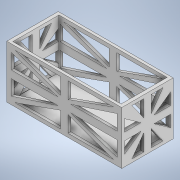
# Autodesk Inventor part: BatteryHolder
Saved by Autodesk Inventor 2022 (Build 260153000, 153)
## iProperties
Created: 2022-02-22
Part Number: BatteryHolder
Material: Generic
Document SubType Name: Modeling
Designer: merky
Density: 1 g/cm^3
Appearance: Default
Author: merky
Autodesk Inventor part; units mm, degrees
ref_plane "YZ Plane" through (0, 0, 0) normal (1, 0, 0) x (0, 1, 0)
ref_plane "XZ Plane" through (0, 0, 0) normal (0, 1, 0) x (-1, 0, 0)
ref_plane "XY Plane" through (0, 0, 0) normal (0, 0, 1) x (1, 0, 0)
sketch "Sketch1" plane through (0, 0, 0) normal (0, 1, 0) x (-1, 0, 0)
  line L0 (-90.805, 38.735) -> (90.805, 38.735)
  line L1 (90.805, 38.735) -> (90.805, -38.735)
  line L2 (90.805, -38.735) -> (-90.805, -38.735)
  line L3 (-90.805, -38.735) -> (-90.805, 38.735)
  line L4 (-90.805, 38.735) -> (90.805, -38.735) construction
  line L5 (90.805, 38.735) -> (-90.805, -38.735) construction
  line L6 (96.52, 43.18) -> (-96.52, 43.18)
  line L7 (-96.52, 43.18) -> (-96.52, -43.18)
  line L8 (-96.52, -43.18) -> (96.52, -43.18)
  line L9 (96.52, -43.18) -> (96.52, 43.18)
  line L10 (96.52, 43.18) -> (-96.52, -43.18) construction
  line L11 (-96.52, 43.18) -> (96.52, -43.18) construction
  point P0 (0, 0)
  dimension "d0" = 181.61
  dimension "d1" = 77.47
  dimension "d2" = 193.04
  dimension "d3" = 86.36
  constraints: 24 end point, 4 midpoint, 4 parallel, 2 horizontal, 2 perpendicular
  measures "d0" distance of L1.end L2.end
  measures "d1" distance of L0.end L1.end
  measures "d2" distance of L8.end L7.end
  measures "d3" distance of L7.end L6.end
extrude "Extrusion1" add sketch "Sketch1" against normal blind 5.08 contours L0 L1 L2 L3 | L9 L8 L7 L6
extrude "Extrusion2" add sketch "Sketch1" along normal blind 83.566
sketch "Sketch2" plane through (-96.52, -5.08, 43.18) normal (0, 0, 1) x (1, 0, 0)
  line L0 (187.325, 88.646) -> (5.715, 88.646) projected
  line L1 (193.04, 88.646) -> (193.04, 0) projected
  line L2 (7.62, 82.423) -> (185.42, 82.423)
  line L3 (185.42, 82.423) -> (185.42, 6.223)
  line L4 (185.42, 6.223) -> (7.62, 6.223)
  line L5 (7.62, 6.223) -> (7.62, 82.423)
  line L6 (185.42, 50.673) -> (185.42, 37.973)
  line L7 (7.62, 37.973) -> (7.62, 50.673)
  line L8 (90.17, 82.423) -> (102.87, 82.423)
  line L9 (102.87, 6.223) -> (90.17, 6.223)
  line L10 (7.62, 50.673) -> (85.5215, 50.673)
  line L11 (107.5185, 50.673) -> (185.42, 50.673)
  line L12 (90.17, 6.223) -> (90.17, 33.3245)
  line L13 (90.17, 55.3215) -> (90.17, 82.423)
  line L14 (185.42, 37.973) -> (107.5185, 37.973)
  line L15 (85.5215, 37.973) -> (7.62, 37.973)
  line L16 (102.87, 82.423) -> (102.87, 55.3215)
  line L17 (102.87, 33.3245) -> (102.87, 6.223)
  arc A0 (90.17, 55.3215) -> (85.5215, 50.673) centre (96.52, 44.323) ccw
  arc A1 (107.5185, 50.673) -> (102.87, 55.3215) centre (96.52, 44.323) ccw
  arc A2 (85.5215, 37.973) -> (90.17, 33.3245) centre (96.52, 44.323) ccw
  arc A3 (102.87, 33.3245) -> (107.5185, 37.973) centre (96.52, 44.323) ccw
  line L18 (7.62, 82.423) -> (13.97, 82.423)
  line L19 (13.97, 82.423) -> (13.97, 76.073)
  line L20 (13.97, 76.073) -> (7.62, 76.073)
  line L21 (7.62, 76.073) -> (7.62, 82.423)
  line L22 (185.42, 82.423) -> (179.07, 82.423)
  line L23 (179.07, 82.423) -> (179.07, 76.073)
  line L24 (179.07, 76.073) -> (185.42, 76.073)
  line L25 (185.42, 76.073) -> (185.42, 82.423)
  line L26 (185.42, 6.223) -> (179.07, 6.223)
  line L27 (179.07, 6.223) -> (179.07, 12.573)
  line L28 (179.07, 12.573) -> (185.42, 12.573)
  line L29 (185.42, 12.573) -> (185.42, 6.223)
  line L30 (7.62, 6.223) -> (13.97, 6.223)
  line L31 (13.97, 6.223) -> (13.97, 12.573)
  line L32 (13.97, 12.573) -> (7.62, 12.573)
  line L33 (7.62, 12.573) -> (7.62, 6.223)
  line L34 (13.97, 6.223) -> (90.17, 33.3245)
  line L35 (85.5215, 37.973) -> (7.62, 12.573)
  line L36 (85.5215, 50.673) -> (7.62, 76.073)
  line L37 (13.97, 82.423) -> (90.17, 55.3215)
  line L38 (102.87, 55.3215) -> (179.07, 82.423)
  line L39 (185.42, 76.073) -> (107.5185, 50.673)
  line L40 (107.5185, 37.973) -> (185.42, 12.573)
  line L41 (179.07, 6.223) -> (102.87, 33.3245)
  point P0 (96.52, 5.08)
  point P1 (96.52, 88.646)
  point P2 (193.04, 44.323)
  point P3 (13.97, 82.423)
  point P4 (13.97, 6.223)
  dimension "d8" = 177.8
  dimension "d9" = 76.2
  dimension "d11" = 12.7
  dimension "d12" = 12.7
  dimension "d13" = 6.35
  dimension "d14" = 6.35
  dimension "d15" = 6.35
  dimension "d16" = 6.35
  dimension "d17" = 6.35
  dimension "d18" = 6.35
  dimension "d19" = 6.35
  dimension "d20" = 6.35
  constraints: 80 end point, 24 parallel, 9 perpendicular, 8 horizontal, 8 point on circle, 4 centre point, 2 midpoint, 2 point on line, 1 coincident
  measures "d8" distance of L3.end L4.end
  measures "d9" distance of L2.end L3.end
  measures "d11" distance of L6.start L6.end
  measures "d12" distance of L9.start L9.end
  measures "d13" distance of L19.end L20.end
  measures "d14" distance of L18.end L19.end
  measures "d15" distance of L24.end L23.end
  measures "d16" distance of L23.end L22.end
  measures "d17" distance of L27.end L28.end
  measures "d18" distance of L26.end L27.end
  measures "d19" distance of L32.end L31.end
  measures "d20" distance of L31.end L30.end
extrude "Extrusion3" cut sketch "Sketch2" against normal through all contours L2 L13 L37 | L36 L10 L5 | L2 L38 L16 | L15 L35 L5 | L39 L3 L11 | L12 L4 L34 | L3 L40 L14 | L17 L41 L4
sketch "Sketch3" plane through (96.52, -5.08, 43.18) normal (1, 0, 0) x (0, 0, -1)
  line L0 (81.915, 88.646) -> (4.445, 88.646) projected
  line L1 (86.36, 0) -> (86.36, 88.646) projected
  line L2 (81.915, 5.08) -> (81.915, 88.646) projected
  line L3 (4.445, 83.058) -> (81.915, 83.058)
  line L4 (81.915, 83.058) -> (81.915, 5.588)
  line L5 (81.915, 5.588) -> (4.445, 5.588)
  line L6 (4.445, 5.588) -> (4.445, 83.058)
  circle A0 centre (43.18, 44.323) radius 12.7
  line L7 (81.915, 50.673) -> (81.915, 37.973)
  line L8 (4.445, 37.973) -> (4.445, 50.673)
  line L9 (36.83, 83.058) -> (49.53, 83.058)
  line L10 (49.53, 5.588) -> (36.83, 5.588)
  line L11 (4.445, 50.673) -> (32.1815, 50.673)
  line L12 (54.1785, 50.673) -> (81.915, 50.673)
  line L13 (36.83, 5.588) -> (36.83, 33.3245)
  line L14 (36.83, 55.3215) -> (36.83, 83.058)
  line L15 (81.915, 37.973) -> (54.1785, 37.973)
  line L16 (32.1815, 37.973) -> (4.445, 37.973)
  line L17 (49.53, 83.058) -> (49.53, 55.3215)
  line L18 (49.53, 33.3245) -> (49.53, 5.588)
  line L19 (4.445, 83.058) -> (17.145, 83.058)
  line L20 (17.145, 83.058) -> (17.145, 70.358)
  line L21 (17.145, 70.358) -> (4.445, 70.358)
  line L22 (4.445, 70.358) -> (4.445, 83.058)
  line L23 (81.915, 83.058) -> (69.215, 83.058)
  line L24 (69.215, 83.058) -> (69.215, 70.358)
  line L25 (69.215, 70.358) -> (81.915, 70.358)
  line L26 (81.915, 70.358) -> (81.915, 83.058)
  line L27 (4.445, 5.588) -> (17.145, 5.588)
  line L28 (17.145, 5.588) -> (17.145, 18.288)
  line L29 (17.145, 18.288) -> (4.445, 18.288)
  line L30 (4.445, 18.288) -> (4.445, 5.588)
  line L31 (81.915, 5.588) -> (69.215, 5.588)
  line L32 (69.215, 5.588) -> (69.215, 18.288)
  line L33 (69.215, 18.288) -> (81.915, 18.288)
  line L34 (81.915, 18.288) -> (81.915, 5.588)
  line L35 (17.145, 5.588) -> (36.83, 33.3245)
  line L36 (32.1815, 37.973) -> (4.445, 18.288)
  line L37 (69.215, 5.588) -> (49.53, 33.3245)
  line L38 (54.1785, 37.973) -> (81.915, 18.288)
  line L39 (49.53, 55.3215) -> (69.215, 83.058)
  line L40 (54.1785, 50.673) -> (81.915, 70.358)
  line L41 (36.83, 55.3215) -> (17.145, 83.058)
  line L42 (32.1815, 50.673) -> (4.445, 70.358)
  point P0 (43.18, 5.08)
  point P1 (43.18, 88.646)
  point P2 (86.36, 44.323)
  dimension "d24" = 25.4
  dimension "d23" = 77.47
  dimension "d25" = 12.7
  dimension "d26" = 12.7
  dimension "d27" = 12.7
  dimension "d28" = 12.7
  dimension "d29" = 12.7
  dimension "d30" = 12.7
  dimension "d31" = 12.7
  dimension "d32" = 12.7
  dimension "d33" = 12.7
  dimension "d34" = 12.7
  constraints: 80 end point, 20 parallel, 15 perpendicular, 8 horizontal, 3 point on line, 2 midpoint, 1 coincident, 10 other
  measures "d23" distance of L3.end L4.end
  measures "d25" distance of L7.start L7.end
  measures "d26" distance of L10.start L10.end
  measures "d27" distance of L20.end L21.end
  measures "d28" distance of L19.end L20.end
  measures "d29" distance of L25.end L24.end
  measures "d30" distance of L24.end L23.end
  measures "d31" distance of L29.end L28.end
  measures "d32" distance of L28.end L27.end
  measures "d33" distance of L32.end L33.end
  measures "d34" distance of L31.end L32.end
extrude "Extrusion4" cut sketch "Sketch3" against normal through all contours L38 L15 L2 | L5 L18 L37 | L12 L40 L2 | L5 L35 L13 | L36 L6 L16 | L17 L3 L39 | L11 L6 L42 | L41 L3 L14
body "Solid1"
